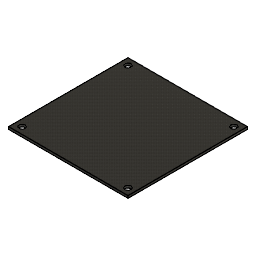
BasePlate (Autodesk Fusion 360 design; units mm, degrees)
Autodesk Fusion 360 part; units mm, degrees
sketch "Sketch1" plane through (0, 0, 0) normal (0, 0, 1) x (1, 0, 0)
  line L0 (101.6, 101.6) -> (-101.6, 101.6)
  line L1 (-101.6, 101.6) -> (-101.6, -101.6)
  line L2 (-101.6, -101.6) -> (101.6, -101.6)
  line L3 (101.6, -101.6) -> (101.6, 101.6)
  line L4 (101.6, 101.6) -> (-101.6, -101.6) construction
  line L5 (-101.6, 101.6) -> (101.6, -101.6) construction
  circle A0 centre (-90, 90) radius 5
  line L6 (0, 0) -> (0, 101.6) construction
  line L7 (0, 0) -> (100, 0) construction
  circle A1 centre (90, 90) radius 5
  circle A2 centre (-90, -90) radius 5
  circle A3 centre (90, -90) radius 5
  dimension "d1" = 203.2
  dimension "d2" = 203.2
  dimension "d3" = 11.6
  constraint horizontal L0
  constraint perpendicular L0 L1
  constraint parallel L0 L2
  constraint parallel L1 L3
  constraint coincident L4 L6.start
  constraint coincident L5 L6.start
  constraint coincident L6.start L7.start
  constraint coincident L5 A0.centre
  constraint midpoint L0 L6.end
  constraint perpendicular L6 L7
  constraint symmetric A0 L6 A1
  constraint symmetric A0 L7 A2
  constraint symmetric L7 A1 A3
  measures "d1" distance of L0.end L1.end
  measures "d2" distance of L1.end L2.end
  measures "d3" horizontal distance of L0.end A0.centre
extrude "Extrude1" add sketch "Sketch1" along normal blind 4
